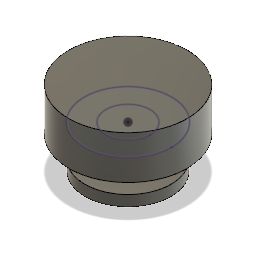
FestingTest v1 (Autodesk Fusion 360 design; units mm, degrees)
Autodesk Fusion 360 part; units mm, degrees
sketch "Sketch1" plane through (0, 0, 0) normal (0, 1, 0) x (1, 0, 0)
  circle A0 centre (0, 0) radius 20
  circle A1 centre (0, 0) radius 10
  dimension "d1" = 40
  dimension "d2" = 20
  constraint coincident A0.centre A1.centre
  measures "d1" diameter of A0
  measures "d2" diameter of A1
extrude "Extrude1" add sketch "Sketch1" along normal blind 5 makes body 1
sketch "Sketch2" plane through (0, 0, 0) normal (0, 1, 0) x (1, 0, 0)
  circle A0 centre (0, 0) radius 10
  circle A1 centre (0, 0) radius 20
  circle A2 centre (0, 0) radius 10
  constraint concentric A0 A2
extrude "Extrude2" add sketch "Sketch2" along normal blind 30 contours A0 A2 bodies 1
sketch "Sketch3" plane through (0, 30, 0) normal (0, 1, 0) x (-1, 0, 0)
  circle A0 centre (0, 0) radius 10
  circle A1 centre (0, 0) radius 20
  dimension "d7" = 40
  constraint coincident A0.centre A1.centre
  measures "d7" diameter of A1
extrude "Extrude3" add sketch "Sketch3" against normal blind 10 bodies 1
ref_plane "WorkPlane1" through (0, 30.1, 0) normal (0, 1, 0) x (1, 0, 0)
sketch "Sketch4" plane through (0, 30.1, 0) normal (0, 1, 0) x (1, 0, 0)
  circle A0 centre (0, 0) radius 27.5
  dimension "d11" = 55
  constraint coincident A0.centre origin
  measures "d11" diameter of A0
extrude "Extrude4" add sketch "Sketch4" along normal blind 5 separate body makes body 2
ref_plane "WorkPlane2" through (0, 30.1, 0) normal (0, -1, 0) x (-1, 0, 0)
sketch "Sketch5" plane through (0, 30.1, 0) normal (0, -1, 0) x (1, 0, 0)
  circle A0 centre (0, 0) radius 20
  circle A1 centre (0, 0) radius 27.5
  circle A2 centre (0, 0) radius 20.1
  circle A3 centre (0, 0) radius 27.5
  dimension "d15" = 40.2
  constraint concentric A0 A2
  constraint concentric A0 A3
  measures "d15" diameter of A2
extrude "Extrude5" add sketch "Sketch5" along normal blind 15 contours A1 A3 bodies 2
ref_plane "WorkPlane3" through (0, 19.9, 0) normal (0, -1, 0) x (1, 0, 0)
sketch "Sketch8" plane through (0, 19.9, 0) normal (0, -1, 0) x (1, 0, 0)
  circle A0 centre (0, 0) radius 10
  circle A1 centre (0, 0) radius 20
  circle A2 centre (0, 0) radius 10.1
  circle A3 centre (0, 0) radius 20.1
  dimension "d20" = 20.2
  dimension "d21" = 40.2
  constraint concentric A0 A2
  constraint concentric A0 A3
  measures "d20" diameter of A2
  measures "d21" diameter of A3
extrude "Extrude8" add sketch "Sketch8" along normal blind 4.9 separate body contours A1 makes body 3
extrude "Extrude9" add sketch "Sketch8" along normal blind 4.9 contours A3 bodies 2 3
extrude "Extrude10" cut 1 faces at (16.6918, 15, -0.9986) along direction (0, 1, 0) blind 0.1 on bodies 2 bodies 2
